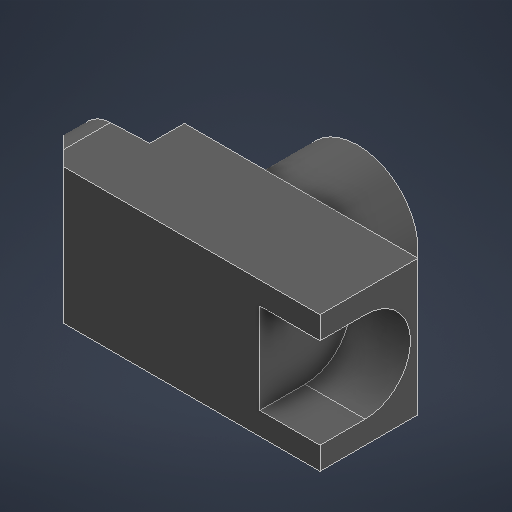
# Autodesk Inventor part: P_handle
Saved by Autodesk Inventor 2026.2 (Build 302298000, 298)
## iProperties
Created: 2025-09-05
Part Number: P_handle
Material: Generisch
Document SubType Name: Modeling
Designer: FAL
Density: 1 g/cm^3
Appearance: Vorgabe
Mass: 1.17123 g
Surface Area: 10.3925 cm^2
Volume: 1.17123 cm^3
Author: FAL
Autodesk Inventor part; units mm, degrees
ref_plane "YZ Plane" through (0, 0, 0) normal (1, 0, 0) x (0, 1, 0)
ref_plane "XZ Plane" through (0, 0, 0) normal (0, 1, 0) x (-1, 0, 0)
ref_plane "XY Plane" through (0, 0, 0) normal (0, 0, 1) x (1, 0, 0)
sketch "Skizze21" plane through (0, 0, 0) normal (0, 0, 1) x (1, 0, 0)
  line L0 (0, 0) -> (20, 0)
  line L1 (20, 0) -> (20, -6.5)
  line L2 (20, -6.5) -> (0, -6.5)
  line L3 (0, -6.5) -> (0, 0)
  dimension "d73" = 6.5
  dimension "d74" = 20
  constraints: 8 end point, 2 perpendicular, 1 horizontal
  measures "d73" distance between parallel lines of L0 L2
  measures "d74" distance between parallel lines of L3 L1
extrude "Extrusion16" add sketch "Skizze21" along normal mid plane 9
sketch "Skizze24" plane through (0, 0, 0) normal (0, 0, 1) x (1, 0, 0)
  line L0 (4.5, -2.3) -> (4.5, 0)
  line L1 (4.5, 0) -> (0, 0)
  line L2 (0, 0) -> (0, -2.5)
  line L3 (20, 0) -> (0, 0) projected
  line L4 (0, 0) -> (0, -6.5) projected
  line L5 (4.5, -2.3) -> (0, -2.5)
  dimension "d92" = 4.5
  dimension "d101" = 2.3
  dimension "d102" = 2.5
  constraints: 8 end point, 2 perpendicular, 1 point on line, 1 vertical
  measures "d92" distance between parallel lines of L2 L0
  measures "d101" distance of L0.start L0.end
  measures "d102" distance of L1.end L2.end
extrude "Extrusion19" cut sketch "Skizze24" along normal mid plane 16.5
sketch "Skizze23" plane through (0, 0, 4.5) normal (0, 1, 0) x (1, 0, 0)
  line L0 (0, 4.5) -> (36.014, 4.5) construction
  circle A0 centre (11, 4.5) radius 4
  line L1 (0, 0) -> (0, 9) projected
  line L2 (4.5, 9) -> (4.5, 0) projected
  dimension "d87" = 8
  dimension "d96" = 6.5
  constraints: 2 end point, 1 centre point, 1 horizontal, 1 point on line
  measures "d87" diameter of A0
  measures "d96" distance from line of L2 A0.centre
extrude "Extrusion18" add sketch "Skizze23" along normal blind 5
chamfer "Fasen2" distance 3 angle 45 1 edges at (0, -6.5, 0)
fillet "Rundung11" radius 2 2 edges at (0, -3, 4.5) (0, -3, -4.5)
sketch "Skizze25" plane through (20, -6.5, 4.5) normal (1, 0, 0) x (0, 0, -1)
  line L0 (9, 6.5) -> (0, 6.5) projected
  line L1 (9, 6.5) -> (9, 0) projected
  circle A0 centre (4.5, 3) radius 3
  line L2 (4.5, 6.5) -> (4.5, 0) construction
  line L3 (9, 0) -> (0, 0) projected
  line L4 (1.5, 3) -> (1.5, 0)
  line L5 (7.5, 0) -> (7.5, 3)
  dimension "d106" = 6
  constraints: 6 end point, 3 point on line, 3 tangent, 2 point on circle, 1 centre point, 1 midpoint, 1 perpendicular, 1 vertical
  measures "d106" diameter of A0
extrude "Extrusion20" cut sketch "Skizze25" against normal blind 4
